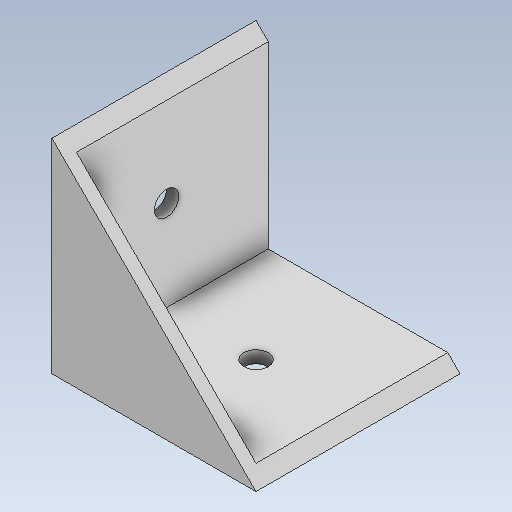
# Autodesk Inventor part: Perfil de unión protección
Saved by Autodesk Inventor 2021 (Build 250183000, 183)
## iProperties
Created: 2021-07-18
Part Number: Perfil de unión protección
Material: Generic
Document SubType Name: Modeling
Designer: maaro
Density: 1 g/cm^3
Appearance: Default
Author: maaro
Autodesk Inventor part; units mm, degrees
ref_plane "YZ Plane" through (0, 0, 0) normal (1, 0, 0) x (0, 1, 0)
ref_plane "XZ Plane" through (0, 0, 0) normal (0, 1, 0) x (-1, 0, 0)
ref_plane "XY Plane" through (0, 0, 0) normal (0, 0, 1) x (1, 0, 0)
sketch "Sketch1" plane through (0, 0, 0) normal (0, 0, 1) x (1, 0, 0)
  line L0 (10, 0) -> (10, 1000) projected
  line L1 (0, 0) -> (1181.712, 0) projected
  line L2 (10, 0) -> (10, 50)
  line L3 (10, 50) -> (60, 0)
  line L4 (10, 50) -> (80.7107, 50) construction
  line L5 (60, 0) -> (10, 0)
  dimension "d0" = 45
  dimension "d1" = 50
  constraints: 8 end point, 2 point on line, 1 collinear, 1 equal length, 1 horizontal
  measures "d0" angle of L3 L4
  measures "d1" distance of L0.start L2.end
extrude "Extrusion1" add sketch "Sketch1" against normal blind 50
shell "Shell1" thickness 3 removed faces 2 at (26.6667, 16.6667, -50) at (43.3333, 16.6667, -16.6667)
sketch "Sketch2" plane through (13, 3, -3) normal (0, 1, 0) x (1, 0, 0)
  circle A0 centre (22, 22) radius 3
  line L0 (47, -3) -> (47, 47) projected
  line L1 (-3, 47) -> (47, -3) construction
  line L2 (-3, -3) -> (47, 47) construction
  point P0 (-13, -3)
  point P1 (22, 22)
  dimension "d5" = 6
  constraints: 4 end point, 1 centre point, 1 coincident, 1 midpoint, 1 perpendicular
  measures "d5" diameter of A0
sketch "Sketch3" plane through (13, 3, -3) normal (1, 0, 0) x (0, 0, -1)
  line L0 (-3, -3) -> (-3, 47) projected
  line L1 (-3, 47) -> (47.1723, -3) construction
  line L2 (47.1723, -3) -> (47.1723, 47.3451)
  line L3 (47.1723, 47.3451) -> (-3, -3) construction
  circle A0 centre (22.0861, 22.1726) radius 3
  point P0 (22.0861, 22.1726)
  dimension "d6" = 6
  constraints: 6 end point, 1 centre point, 1 coincident, 1 midpoint, 1 parallel, 1 perpendicular
  measures "d6" diameter of A0
extrude "Extrusion2" cut sketch "Sketch2" against normal through all
extrude "Extrusion3" cut sketch "Sketch3" against normal through all
body "Solid1"
